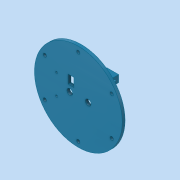
# Autodesk Inventor part: foreElectronicsSealingWallRear
Saved by Autodesk Inventor 2017 (Build 210142000, 142)
## iProperties
Created: 2016-12-09
Part Number: foreElectronicsSealingWallRear
Material: ABS Plastic
Document SubType Name: Modeling
Designer: techn
Density: 1.06 g/cm^3
Appearance: Sky Blue Dark
Mass: 27.6637 g
Surface Area: 174.765 cm^2
Volume: 26.0979 cm^3
Author: techn
Autodesk Inventor part; units mm, degrees
ref_plane "YZ Plane" through (0, 0, 0) normal (1, 0, 0) x (0, 1, 0)
ref_plane "XZ Plane" through (0, 0, 0) normal (0, 1, 0) x (-1, 0, 0)
ref_plane "XY Plane" through (0, 0, 0) normal (0, 0, 1) x (1, 0, 0)
sketch "Sketch1" plane through (0, 0, 0) normal (0, 0, 1) x (1, 0, 0)
  circle A0 centre (0, 0) radius 47.625
  line L0 (0, 0) -> (0, 41.91)
  line L1 (0, 0) -> (41.91, 0) construction
  circle A1 centre (0, 41.91) radius 1.8415
  circle A2 centre (-36.2951, 20.955) radius 1.8415
  circle A3 centre (-36.2951, -20.955) radius 1.8415
  circle A4 centre (0, -41.91) radius 1.8415
  circle A5 centre (36.2951, -20.955) radius 1.8415
  circle A6 centre (36.2951, 20.955) radius 1.8415
  dimension "d0" = 95.25
  dimension "d1" = 41.91
  dimension "d2" = 90
  dimension "d3" = 3.683
  dimension "d6" = 360
  constraints: 7 centre point, 4 end point, 2 coincident, 1 horizontal, 1 perpendicular, 1 vertical, 13 other
  measures "d0" diameter of A0
  measures "d1" distance of L0.start L0.end
  measures "d2" angle of L1 L0
  measures "d3" diameter of A1
extrude "Extrusion1" add sketch "Sketch1" along normal blind 3.175
sketch "Sketch2" plane through (0, 0, 0) normal (0, 0, -1) x (-1, 0, 0)
  line L0 (-18.415, 17.399) -> (-5.715, 17.399)
  line L1 (-5.715, 17.399) -> (-5.715, 9.779)
  line L2 (-5.715, 9.779) -> (-18.415, 9.779)
  line L3 (-18.415, 9.779) -> (-18.415, 17.399)
  line L4 (-18.415, -30.861) -> (-5.715, -30.861)
  line L5 (-5.715, -30.861) -> (-5.715, -38.481)
  line L6 (-5.715, -38.481) -> (-18.415, -38.481)
  line L7 (-18.415, -38.481) -> (-18.415, -30.861)
  point P0 (0, 0)
  dimension "d10" = 40.64
  dimension "d11" = 9.779
  dimension "d12" = 7.62
  dimension "d13" = 7.62
  dimension "d14" = 12.7
  dimension "d31" = 5.715
  constraints: 16 end point, 4 parallel, 2 horizontal, 2 perpendicular, 2 point on line
  measures "d10" distance between parallel lines of L4 L2
  measures "d11" distance from line of point (0, 0) L2
  measures "d12" distance between parallel lines of L0 L2
  measures "d13" distance between parallel lines of L4 L6
  measures "d14" distance of L0.start L0.end
  measures "d31" distance from line of L1 point (0, 0)
extrude "Extrusion2" add sketch "Sketch2" along normal blind 22.225
sketch "Sketch3" plane through (0, 0, 3.175) normal (0, 0, 1) x (1, 0, 0)
  line L0 (-11.1125, 15.875) -> (-4.7625, 15.875)
  line L1 (-4.7625, 15.875) -> (-4.7625, 6.35)
  line L2 (-4.7625, 6.35) -> (-11.1125, 6.35)
  line L3 (-11.1125, 6.35) -> (-11.1125, 15.875)
  point P0 (0, 0)
  dimension "d18" = 6.35
  dimension "d19" = 9.525
  dimension "d33" = 4.7625
  dimension "d34" = 6.35
  constraints: 8 end point, 2 parallel, 1 horizontal, 1 perpendicular
  measures "d18" distance of L1.end L2.end
  measures "d19" distance of L2.end L0.start
  measures "d33" distance from line of point (0, 0) L1
  measures "d34" distance from line of point (0, 0) L2
extrude "Extrusion3" cut sketch "Sketch3" against normal blind 19.05
sketch "Sketch4" plane through (5.715, -38.481, 0) normal (-1, 0, 0) x (0, 0, 1)
  line L0 (0, 7.62) -> (0, 0) projected
  line L1 (0, 7.62) -> (-22.225, 7.62) projected
  line L2 (-22.225, 0) -> (-22.225, 7.62) projected
  line L3 (0, 0) -> (-22.225, 0) projected
  circle A0 centre (-17.78, 3.81) radius 1.27
  circle A1 centre (-7.62, 3.81) radius 1.27
  line L4 (0, 7.62) -> (-22.225, 7.62) projected
  line L5 (0, 55.88) -> (0, 48.26) projected
  line L6 (0, 55.88) -> (-22.225, 55.88) projected
  line L7 (-22.225, 48.26) -> (-22.225, 55.88) projected
  line L8 (0, 48.26) -> (-22.225, 48.26) projected
  circle A2 centre (-17.78, 52.07) radius 1.27
  circle A3 centre (-7.62, 52.07) radius 1.27
  point P0 (0, 38.481)
  dimension "d22" = 2.54
  dimension "d23" = 2.54
  dimension "d24" = 3.81
  dimension "d25" = 10.16
  dimension "d27" = 2.54
  dimension "d28" = 2.54
  dimension "d32" = 4.445
  constraints: 4 centre point
  measures "d22" diameter of A0
  measures "d23" diameter of A1
  measures "d24" distance from line of L1 A0.centre
  measures "d25" distance of A1.centre A0.centre
  measures "d27" diameter of A2
  measures "d28" diameter of A3
  measures "d32" distance from line of A0.centre L2
extrude "Extrusion4" cut sketch "Sketch4" against normal blind 19.05 contours A0 | A1 | A2 | A3
sketch "Sketch5" plane through (0, 0, 0) normal (0, 0, -1) x (-1, 0, 0)
  circle A0 centre (23.495, 11.1125) radius 1.143
  circle A1 centre (23.495, -11.1125) radius 1.143
  point P0 (0, 0)
  dimension "d35" = 2.286
  dimension "d36" = 2.286
  dimension "d37" = 22.225
  dimension "d38" = 11.1125
  dimension "d39" = 23.495
  constraints: 2 centre point
  measures "d35" diameter of A0
  measures "d36" diameter of A1
  measures "d37" distance of A1.centre A0.centre
  measures "d38" vertical distance of point (0, 0) A0.centre
  measures "d39" horizontal distance of A0.centre point (0, 0)
extrude "Extrusion5" cut sketch "Sketch5" against normal blind 25.4
sketch "Sketch8" plane through (0, 0, 0) normal (0, 0, -1) x (-1, 0, 0)
  circle A0 centre (23.495, 11.1125) radius 1.143 projected
  circle A1 centre (23.495, -11.1125) radius 1.143 projected
  line L0 (11.1125, 15.875) -> (11.1125, 6.35) projected
  line L1 (11.1125, 6.35) -> (4.7625, 6.35) projected
  line L2 (4.7625, 6.35) -> (4.7625, 15.875) projected
  line L3 (4.7625, 15.875) -> (11.1125, 15.875) projected
  line L4 (-5.715, 17.399) -> (-5.715, 9.779) projected
  line L5 (-5.715, 9.779) -> (-18.415, 9.779) projected
  line L6 (-18.415, 9.779) -> (-18.415, 17.399) projected
  line L7 (-18.415, 17.399) -> (-5.715, 17.399) projected
  line L8 (-5.715, -30.861) -> (-5.715, -38.481) projected
  line L9 (-5.715, -38.481) -> (-18.415, -38.481) projected
  line L10 (-18.415, -38.481) -> (-18.415, -30.861) projected
  line L11 (-18.415, -30.861) -> (-5.715, -30.861) projected
  circle A2 centre (-36.2951, 20.955) radius 1.8415 projected
  circle A3 centre (-36.2951, -20.955) radius 1.8415 projected
  circle A4 centre (0, -41.91) radius 1.8415 projected
  circle A5 centre (36.2951, -20.955) radius 1.8415 projected
  circle A6 centre (36.2951, 20.955) radius 1.8415 projected
  circle A7 centre (0, 41.91) radius 1.8415 projected
  circle A8 centre (0, 0) radius 47.625 projected
  circle A9 centre (9.2075, 0) radius 3.175
  circle A10 centre (-10.7925, 0) radius 3.175
  dimension "d42" = 6.35
  dimension "d43" = 6.35
  dimension "d44" = 1.905
  dimension "d45" = 6.35
  dimension "d46" = 20
  constraints: 2 centre point
  measures "d42" diameter of A9
  measures "d43" distance from line of L1 A9.centre
  measures "d44" distance from line of A9.centre L0
  measures "d45" diameter of A10
  measures "d46" distance of A10.centre A9.centre
extrude "Extrusion6" cut sketch "Sketch8" against normal blind 25.4 contours A9 | A10
equation "\"d38\" = 0.5 * d37"
body "Solid1"
